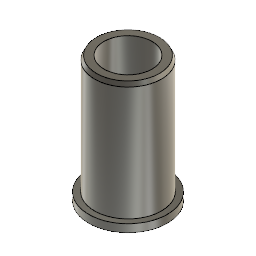
auger-bearing-bushing (Autodesk Fusion 360 design; units mm, degrees)
Autodesk Fusion 360 part; units mm, degrees
sketch "Sketch1" plane through (0, 0, 0) normal (0, 0, 1) x (1, 0, 0)
  circle A0 centre (0, 0) radius 10
  dimension "d1" = 20
  measures "d1" diameter of A0
extrude "Extrude1" add sketch "Sketch1" along normal blind 2
sketch "Sketch2" plane through (0, 0, 2) normal (0, 0, 1) x (-1, 0, 0)
  circle A0 centre (0, 0) radius 10
  circle A1 centre (0, 0) radius 8.5
  dimension "d4" = 17
  measures "d4" diameter of A1
extrude "Extrude2" add sketch "Sketch2" along normal blind 30 contours A1
sketch "Sketch3" plane through (0, 0, 32) normal (0, 0, 1) x (-1, 0, 0)
  circle A0 centre (0, 0) radius 8.5
  circle A1 centre (0, 0) radius 6.1
  dimension "d7" = 12.2
  measures "d7" diameter of A1
extrude "Extrude3" cut sketch "Sketch3" against normal blind 60 contours A1
chamfer "Chamfer1" distance 0.5 distance2 1 2 edges at (5.6872, 2.2059, 0) (7.9248, 3.0737, 32) measured on face at (8.6401, -0.7999, 0) measured on face at (-7.6684, 0.4223, 32)
